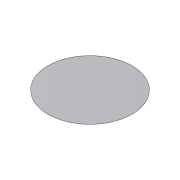
# Autodesk Inventor part: Exp1_extramass
Saved by Autodesk Inventor 2014 SP1 (Build 180222100, 222)
## iProperties
Created: 2014-07-15
Part Number: Exp1_extramass
Material: Aluminum 6061
Document SubType Name: Modeling
Designer: RDavis
Mass: 5.95481 g
Surface Area: 142.69 cm^2
Volume: 2.19735 cm^3
Density: 2.71 g/cm^3
Appearance: Aluminum - Flat
Author: RDavis
Autodesk Inventor part; units mm, degrees
ref_plane "YZ Plane" through (0, 0, 0) normal (1, 0, 0) x (0, 1, 0)
ref_plane "XZ Plane" through (0, 0, 0) normal (0, 1, 0) x (-1, 0, 0)
ref_plane "XY Plane" through (0, 0, 0) normal (0, 0, 1) x (1, 0, 0)
sketch "Sketch1" plane through (0, 0, 0) normal (0, 0, 1) x (1, 0, 0)
  circle A0 centre (0, 0) radius 47.5
  dimension "d0" = 95
  constraints: 1 centre point, 1 coincident
  measures "d0" diameter of A0
extrude "Extrusion1" add sketch "Sketch1" along normal blind 0.1
body "Solid1"
